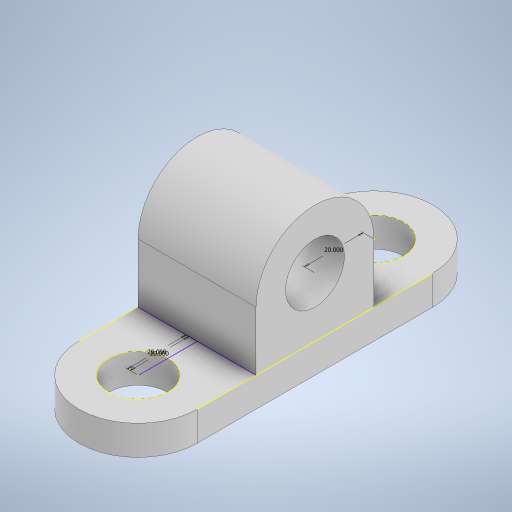
# Autodesk Inventor part: Tarea No 1 - 1053321
Saved by Autodesk Inventor 2024 (Build 280153000, 153)
## iProperties
Created: 2024-02-05
Material: Generic
Document SubType Name: Modeling
Density: 1 g/cm^3
Appearance: Default
Part Number: Tarea No 1 - 1053321
Author: Rodrigo Ochoa
Title: Tarea 1
Autodesk Inventor part; units mm, degrees
ref_plane "YZ Plane" through (0, 0, 0) normal (1, 0, 0) x (0, 1, 0)
ref_plane "XZ Plane" through (0, 0, 0) normal (0, 1, 0) x (-1, 0, 0)
ref_plane "XY Plane" through (0, 0, 0) normal (0, 0, 1) x (1, 0, 0)
sketch "Sketch1" plane through (0, 0, 0) normal (0, 1, 0) x (-1, 0, 0)
  line L0 (6.704, 12.1536) -> (6.704, -2019.8464)
  line L1 (-1009.296, -2019.8464) -> (-1009.296, 12.1536)
  arc A0 (6.704, 12.1536) -> (-1009.296, 12.1536) centre (-501.296, 12.1536) ccw
  arc A1 (-1009.296, -2019.8464) -> (6.704, -2019.8464) centre (-501.296, -2019.8464) ccw
  circle A2 centre (-501.296, 12.1536) radius 254
  circle A3 centre (-501.296, -2019.8464) radius 254
  point P0 (0, 0)
  dimension "d0" = 2032
  dimension "d1" = 1016
  dimension "d2" = 2032
  dimension "d3" = 508
  dimension "d4" = 508
  constraints: 4 centre point, 4 end point, 4 point on circle, 2 coincident, 1 vertical
  measures "d0" distance of L0.start L0.end
  measures "d1" distance of L0.end L1.start
  measures "d2" distance of L1.start L1.end
  measures "d3" diameter of A2
  measures "d4" diameter of A3
extrude "Extrusion1" add sketch "Sketch1" along normal blind 254
sketch "Sketch2" plane through (0, 254, 0) normal (0, 1, 0) x (1, 0, 0)
  circle A0 centre (501.296, -12.1536) radius 254 projected
  line L0 (501.296, 495.8464) -> (0, 495.8464)
  line L1 (501.296, 495.8464) -> (1009.296, 495.8464)
  line L2 (1009.296, -12.1536) -> (1009.296, 2019.8464) projected
  circle A1 centre (501.296, 2019.8464) radius 254 projected
  line L3 (501.296, 1511.8464) -> (-6.704, 1511.8464)
  line L4 (-6.704, 2019.8464) -> (-6.704, -12.1536) projected
  line L5 (501.296, 1511.8464) -> (1009.296, 1511.8464)
  point P0 (0, 0)
  dimension "d9" = 508
  dimension "d10" = 508
  constraints: 8 end point, 3 point on line, 1 horizontal, 1 perpendicular
  measures "d9" distance of A0.centre L0.start
  measures "d10" distance of A1.centre L3.start
sketch "Sketch3" plane through (0, 254, 0) normal (0, 1, 0) x (1, 0, 0)
  point P0 (0, 0)
sketch "Sketch4" plane through (0, 254, 0) normal (0, 1, 0) x (1, 0, 0)
  line L0 (502.0713, -12.1292) -> (502.0713, 495.8708)
  line L1 (502.0713, 495.8708) -> (-6.704, 495.8708)
  line L2 (-6.704, 2019.8464) -> (-6.704, -12.1536) projected
  point P0 (0, 0)
  dimension "d11" = 508
  constraints: 4 end point, 1 perpendicular, 1 point on line, 1 vertical
  measures "d11" distance of L0.start L0.end
sketch "Sketch5" plane through (0, 254, 0) normal (0, 1, 0) x (1, 0, 0)
  point P0 (0, 0)
sketch "Sketch6" plane through (0, 254, 0) normal (0, 1, 0) x (1, 0, 0)
  point P0 (0, 0)
sketch "Sketch7" plane through (0, 254, 0) normal (0, 1, 0) x (1, 0, 0)
  point P0 (0, 0)
sketch "Sketch8" plane through (0, 254, 0) normal (0, 1, 0) x (1, 0, 0)
  point P0 (0, 0)
sketch "Sketch9" plane through (0, 0, 0) normal (0, -1, 0) x (1, 0, 0)
  point P0 (0, 0)
sketch "Sketch10" plane through (1009.296, 0, 12.1536) normal (1, 0, 0) x (0, 0, -1)
  line L0 (0, 254) -> (-508, 254) projected
  line L1 (0, 254) -> (508, 254)
  line L2 (2032, 254) -> (0, 254) projected
  line L3 (508, 254) -> (508, 762)
  line L4 (1524, 762) -> (1524, 254)
  line L5 (1524, 254) -> (508, 254)
  arc A0 (1524, 762) -> (508, 762) centre (1016, 762) ccw
  circle A1 centre (1016, 762) radius 254
  point P0 (12.1536, 0)
  dimension "d12" = 508
  dimension "d13" = 508
  dimension "d14" = 1016
  dimension "d15" = 508
  dimension "d16" = 508
  constraints: 8 end point, 2 centre point, 2 point on circle, 2 point on line, 1 coincident, 1 perpendicular
  measures "d12" distance of L0.start L1.end
  measures "d13" distance of L1.end L3.end
  measures "d14" distance of L4.start L3.end
  measures "d15" distance of L4.start L4.end
  measures "d16" diameter of A1
extrude "Extrusion2" add sketch "Sketch10" against normal blind 1016
body "Solid1"
